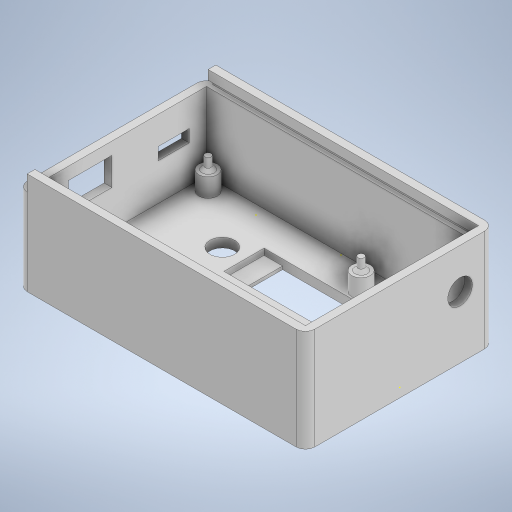
# Autodesk Inventor part: bt-case
Saved by Autodesk Inventor 2024.2 (Build 282272000, 272)
## iProperties
Created: 2025-05-09
Part Number: bt-case
Material: Типовые
Document SubType Name: Modeling
Designer: nikit
Density: 1 g/cm^3
Appearance: По умолчанию
Author: nikit
Autodesk Inventor part; units mm, degrees
ref_plane "YZ Plane" through (0, 0, 0) normal (1, 0, 0) x (0, 1, 0)
ref_plane "XZ Plane" through (0, 0, 0) normal (0, 1, 0) x (-1, 0, 0)
ref_plane "XY Plane" through (0, 0, 0) normal (0, 0, 1) x (1, 0, 0)
sketch "Эскиз1" plane through (0, 0, 0) normal (0, 1, 0) x (-1, 0, 0)
  line L0 (43.5, -27.5) -> (-43.5, -27.5)
  line L1 (-43.5, -27.5) -> (-43.5, 27.5)
  line L2 (-43.5, 27.5) -> (43.5, 27.5)
  line L3 (43.5, 27.5) -> (43.5, -27.5)
  line L4 (43.5, -27.5) -> (-43.5, 27.5) construction
  line L5 (-43.5, -27.5) -> (43.5, 27.5) construction
  arc A0 (46.5, 27.5) -> (43.5, 30.5) centre (43.5, 27.5) ccw
  line L6 (43.5, -30.5) -> (-43.5, -30.5)
  line L7 (-46.5, -27.5) -> (-46.5, 27.5)
  line L8 (-43.5, 30.5) -> (43.5, 30.5)
  line L9 (46.5, 27.5) -> (46.5, -27.5)
  arc A1 (43.5, -30.5) -> (46.5, -27.5) centre (43.5, -27.5) ccw
  arc A2 (-46.5, -27.5) -> (-43.5, -30.5) centre (-43.5, -27.5) ccw
  arc A3 (-43.5, 30.5) -> (-46.5, 27.5) centre (-43.5, 27.5) ccw
  point P0 (0, 0)
  dimension "d0" = 87
  dimension "d1" = 55
  dimension "d4" = 6
  constraints: 20 end point, 8 point on circle, 5 tangent, 4 centre point, 4 coincident, 2 midpoint, 2 parallel, 2 perpendicular, 1 horizontal
  measures "d0" distance of L1.end L2.end
  measures "d1" distance of L0.end L1.end
  measures "d4" diameter of A0
extrude "Выдавливание1" add sketch "Эскиз1" along normal blind 25
sketch "Эскиз2" plane through (0, 0, 0) normal (0, -1, 0) x (1, 0, 0)
  line L0 (43.5, -27.5) -> (43.5, 27.5) projected
  circle A0 centre (43.5, -27.5) radius 3
  line L1 (-43.5, -27.5) -> (43.5, -27.5) projected
  circle A1 centre (-43.5, -27.5) radius 3
  line L2 (43.5, 27.5) -> (-43.5, 27.5) projected
  circle A2 centre (-43.5, 27.5) radius 3
  circle A3 centre (43.5, 27.5) radius 3
  line L3 (-43.5, -30.5) -> (43.5, -30.5)
  line L4 (46.5, 27.5) -> (46.5, -27.5) projected
  line L5 (46.5, -27.5) -> (46.5, 27.5)
  line L6 (-43.5, 30.5) -> (43.5, 30.5) projected
  line L7 (43.5, 30.5) -> (-43.5, 30.5)
  line L8 (-46.5, 27.5) -> (-46.5, -27.5)
  point P0 (0, 0)
  constraints: 8 end point, 5 point on circle, 5 tangent, 4 centre point, 2 collinear, 1 coincident
extrude "Выдавливание2" add sketch "Эскиз2" along normal blind 3
sketch "Эскиз3" plane through (0, 0, 0) normal (0, 1, 0) x (1, 0, 0)
  line L0 (43.5, 27.5) -> (43.5, -27.5) projected
  line L1 (-43.5, 27.5) -> (43.5, 27.5) projected
  line L2 (21.4, 27.5) -> (38.4, 27.5) construction
  circle A0 centre (21.4, 10.5) radius 3.5
  circle A1 centre (21.4, 10.5) radius 4
  point P0 (0, 0)
  dimension "d15" = 8
  constraints: 2 centre point, 2 end point, 1 coincident, 1 horizontal, 1 point on line
  measures "d15" diameter of A1
extrude "Выдавливание3" cut sketch "Эскиз3" against normal blind 86.25 contours A0 | A1
sketch "Эскиз4" plane through (0, 0, 0) normal (0, 1, 0) x (1, 0, 0)
  circle A0 centre (21.4, 10.5) radius 4 projected
  line L0 (21.4, 10.5) -> (14.4, 10.5)
  line L1 (14.4, 10.5) -> (-23.6, 10.5)
  line L2 (14.4, 10.5) -> (8.4, 10.5)
  line L3 (8.4, 10.5) -> (-18.6, 10.5)
  line L4 (8.4, 16.5) -> (-18.6, 16.5)
  line L5 (-18.6, 16.5) -> (-18.6, 4.5)
  line L6 (-18.6, 4.5) -> (8.4, 4.5)
  line L7 (8.4, 4.5) -> (8.4, 16.5)
  line L8 (8.4, 16.5) -> (-18.6, 4.5) construction
  line L9 (-18.6, 16.5) -> (8.4, 4.5) construction
  line L10 (-23.6, 4.5) -> (14.4, 4.5)
  line L11 (14.4, 4.5) -> (14.4, 16.5)
  line L12 (14.4, 16.5) -> (-23.6, 16.5)
  line L13 (-23.6, 16.5) -> (-23.6, 4.5)
  point P0 (0, 0)
  point P1 (-5.1, 10.5)
  dimension "d18" = 7
  dimension "d19" = 38
  dimension "d20" = 6
  dimension "d21" = 27
  dimension "d22" = 12
  constraints: 28 end point, 4 parallel, 3 horizontal, 3 midpoint, 3 point on line, 2 perpendicular
  measures "d18" distance of L0.start L0.end
  measures "d19" distance of L0.end L1.end
  measures "d20" distance of L0.end L2.end
  measures "d21" distance of L2.end L3.end
  measures "d22" distance of L5.end L4.end
extrude "Выдавливание4" cut sketch "Эскиз4" against normal blind 2 contours L11 L10 L7 L1 | L1 L7 L12 L11 | L5 L10 L13 L1 | L1 L13 L12 L5
sketch "Эскиз5" plane through (0, 0, 0) normal (0, 1, 0) x (1, 0, 0)
  line L0 (8.4, 4.5) -> (8.4, 16.5) projected
  line L1 (-23.6, 16.5) -> (-18.6, 16.5) projected
  line L2 (8.4, 4.5) -> (-18.6, 4.5)
  line L3 (-18.6, 4.5) -> (-18.6, 16.5)
  line L4 (-18.6, 16.5) -> (8.4, 16.5)
  line L5 (8.4, 16.5) -> (8.4, 4.5)
  point P0 (0, 0)
  constraints: 8 end point, 2 parallel, 1 horizontal, 1 perpendicular
extrude "Выдавливание5" cut sketch "Эскиз5" against normal blind 3
sketch "Эскиз6" plane through (0, 0, 0) normal (0, 1, 0) x (1, 0, 0)
  point P0 (0, 0)
sketch "Эскиз7" plane through (0, 0, 0) normal (0, 1, 0) x (1, 0, 0)
  line L0 (-43.5, 27.5) -> (43.5, 27.5) projected
  line L1 (43.5, 27.5) -> (39.5, 27.5)
  line L2 (39.5, 27.5) -> (39.5, 24)
  line L3 (39.5, 24) -> (43.5, 24)
  line L4 (43.5, 24) -> (43.5, 27.5)
  circle A0 centre (39.5, 24) radius 3
  line L5 (-43.5, -27.5) -> (-43.5, 27.5) projected
  line L6 (-43.5, -27.5) -> (-39.5, -27.5)
  line L7 (-39.5, -27.5) -> (-39.5, -23)
  line L8 (-39.5, -23) -> (-43.5, -23)
  line L9 (-43.5, -23) -> (-43.5, -27.5)
  circle A1 centre (-39.5, -23) radius 3
  arc A2 (-43.5, 30.5) -> (-46.5, 27.5) centre (-43.5, 27.5) ccw projected
  line L10 (-43.5, 27.5) -> (-13.5, 27.5)
  line L11 (-13.5, 27.5) -> (-13.5, 20.5)
  line L12 (-13.5, 20.5) -> (-43.5, 20.5)
  line L13 (-43.5, 20.5) -> (-43.5, 27.5)
  circle A3 centre (-13.5, 20.5) radius 3
  point P0 (0, 0)
  dimension "d27" = 4
  dimension "d28" = 3.5
  dimension "d29" = 6
  dimension "d30" = 4
  dimension "d31" = 4.5
  dimension "d32" = 6
  dimension "d33" = 30
  dimension "d34" = 7
  dimension "d35" = 6
  constraints: 24 end point, 6 parallel, 3 centre point, 3 coincident, 3 horizontal, 3 perpendicular
  measures "d27" distance of L3.end L2.end
  measures "d28" distance of L2.end L1.end
  measures "d29" diameter of A0
  measures "d30" distance of L8.end L7.end
  measures "d31" distance of L7.end L6.end
  measures "d32" diameter of A1
  measures "d33" distance of L11.end L12.end
  measures "d34" distance of L10.end L11.end
  measures "d35" diameter of A3
extrude "Выдавливание6" add sketch "Эскиз7" along normal blind 6 contours A3 L12 L11 | L11 L12 A3 | A0 L3 L2 | L2 L3 A0 | A1 L7 L8 | L8 L7 A1
sketch "Эскиз8" plane through (39.5, 6, -24) normal (0, 1, 0) x (1, 0, 0)
  circle A0 centre (0, 0) radius 3 projected
  circle A1 centre (0, 0) radius 1
  circle A2 centre (-53, -3.5) radius 3 projected
  circle A3 centre (-53, -3.5) radius 1
  circle A4 centre (-79, -47) radius 3 projected
  circle A5 centre (-79, -47) radius 1
  point P0 (-39.5, -24)
  dimension "d38" = 2
  dimension "d39" = 2
  dimension "d40" = 2
  constraints: 3 centre point, 3 coincident
  measures "d38" diameter of A1
  measures "d39" diameter of A3
  measures "d40" diameter of A5
extrude "Выдавливание7" add sketch "Эскиз8" along normal blind 4 contours A1 | A3 | A5
chamfer "Фаска1" distance 1 angle 45 3 edges at (-40.5, 6, 23) (38.5, 6, -24) (-14.5, 6, -20.5)
sketch "Эскиз9" plane through (-43.5, 25, 27.5) normal (1, 0, 0) x (0, 0, -1)
  point P0 (27.5, -25)
sketch "Эскиз10" plane through (-43.5, 25, 27.5) normal (1, 0, 0) x (0, 0, -1)
  point P0 (27.5, -25)
sketch "Эскиз11" plane through (-43.5, 25, 27.5) normal (1, 0, 0) x (0, 0, -1)
  line L0 (55, 0) -> (55, -28) projected
  line L1 (55, -25) -> (45, -25)
  line L2 (45, -25) -> (45, -15)
  line L3 (45, -15) -> (55, -15)
  line L4 (55, -15) -> (55, -25)
  circle A0 centre (45, -15) radius 6.5
  point P0 (27.5, -25)
  dimension "d54" = 10
  dimension "d55" = 10
  dimension "d56" = 13
  constraints: 8 end point, 2 parallel, 1 centre point, 1 coincident, 1 horizontal, 1 perpendicular, 1 point on line
  measures "d54" distance of L2.end L3.end
  measures "d55" distance of L1.end L2.end
  measures "d56" diameter of A0
extrude "Выдавливание8" cut sketch "Эскиз11" against normal blind 5.75 contours A0 L2 L3 | L3 L2 A0
sketch "Эскиз12" plane through (46.5, 25, 27.5) normal (1, 0, 0) x (0, 0, -1)
  line L0 (-3, -28) -> (0, -28) projected
  line L1 (0, -28) -> (0, -25)
  line L2 (0, -28) -> (0, 0) projected
  line L3 (0, -25) -> (0, -17)
  line L4 (6.5, -19) -> (2.5, -19) projected
  line L5 (14.25, -17) -> (14.25, -20.5)
  line L6 (5, -20.5) -> (23.5, -20.5)
  line L7 (23.5, -20.5) -> (23.5, -17)
  line L8 (5, -17) -> (5, -20.5)
  line L9 (5, -20.5) -> (23.5, -17) construction
  line L10 (23.5, -20.5) -> (5, -17) construction
  line L11 (5, -17) -> (23.5, -17)
  point P0 (27.5, -25)
  point P1 (14.25, -18.75)
  dimension "d72" = 3.5
  dimension "d73" = 18.5
  constraints: 18 end point, 3 midpoint, 2 horizontal, 2 point on line, 1 parallel, 1 perpendicular, 1 vertical
  measures "d72" distance of L5.start L5.end
  measures "d73" distance of L6.start L6.end
extrude "Выдавливание9" cut sketch "Эскиз12" against normal blind 4.25
sketch "Эскиз13" plane through (0, 25, 0) normal (0, 1, 0) x (1, 0, 0)
  point P0 (0, 0)
sketch "Эскиз14" plane through (0, 25, 0) normal (0, 1, 0) x (1, 0, 0)
  line L0 (-43.5, 27.5) -> (43.5, 27.5) projected
  line L1 (43.5, 27.5) -> (-43.5, 27.5)
  line L2 (-43.5, 27.5) -> (-43.5, -27.5)
  line L3 (-43.5, -27.5) -> (43.5, -27.5)
  arc A0 (46.5, 27.5) -> (43.5, 30.5) centre (43.5, 27.5) ccw projected
  line L4 (43.5, 27.5) -> (43.5, 30.5)
  line L5 (43.5, 30.5) -> (-43.5, 30.5)
  arc A1 (-46.5, -27.5) -> (-43.5, -30.5) centre (-43.5, -27.5) ccw projected
  line L6 (-43.5, -30.5) -> (43.5, -30.5)
  line L7 (43.5, -30.5) -> (43.5, -27.5)
  arc A2 (-46.5, -27.5) -> (-43.5, -30.5) centre (-43.5, -27.5) ccw
  arc A3 (-43.5, 30.5) -> (-46.5, 27.5) centre (-43.5, 27.5) ccw projected
  arc A4 (-43.5, 30.5) -> (-46.5, 27.5) centre (-43.5, 27.5) ccw
  line L8 (-46.5, 27.5) -> (-46.5, -27.5)
  point P0 (0, 0)
  constraints: 16 end point, 5 point on circle, 5 tangent, 4 perpendicular, 2 centre point, 2 vertical, 1 collinear, 1 horizontal
extrude "Выдавливание10" add sketch "Эскиз14" along normal blind 5
sketch "Эскиз15" plane through (43.5, 25, 30.5) normal (1, 0, 0) x (0, 0, -1)
  line L0 (3, 0) -> (3, 5) projected
  line L1 (3, 0) -> (1, 0)
  line L2 (1, 0) -> (1, 2)
  line L3 (1, 2) -> (3, 2)
  line L4 (3, 2) -> (3, 0)
  line L5 (61, 0) -> (58, 0) projected
  line L6 (58, 0) -> (60, 0)
  line L7 (60, 0) -> (60, 2)
  line L8 (60, 2) -> (58, 2)
  line L9 (58, 2) -> (58, 0)
  point P0 (30.5, -25)
  point P1 (3, 2)
  dimension "d78" = 2
  dimension "d79" = 2
  dimension "d80" = 2
  dimension "d81" = 2
  constraints: 16 end point, 4 parallel, 2 horizontal, 2 perpendicular
  measures "d78" distance of L2.end L3.end
  measures "d79" distance of L1.end L2.end
  measures "d80" distance of L8.end L7.end
  measures "d81" distance of L7.end L6.end
extrude "Выдавливание11" cut sketch "Эскиз15" against normal blind 87
mirror "Зеркальное отражение1" about plane through (0, 0, 0) normal (1, 0, 0) remove original yes
sketch "Эскиз16" plane through (-43.5, 0, -27.5) normal (0, 1, 0) x (1, 0, 0)
  line L0 (29.1, -11) -> (29.1, -23) projected
  line L1 (29.1, -11) -> (29.1, -10.5)
  line L2 (62.1, -23) -> (67.1, -23) projected
  line L3 (67.1, -23) -> (67.1, -23.5)
  line L4 (29.1, -10.5) -> (67.1, -10.5)
  line L5 (67.1, -10.5) -> (67.1, -23.5)
  line L6 (67.1, -23.5) -> (29.1, -23.5)
  line L7 (29.1, -23.5) -> (29.1, -10.5)
  point P0 (43.5, -27.5)
  dimension "d84" = 0.5
  dimension "d85" = 0.5
  constraints: 12 end point, 2 parallel, 2 vertical, 1 horizontal, 1 perpendicular
  measures "d84" distance of L0.start L1.end
  measures "d85" distance of L2.end L3.end
extrude "Выдавливание12" cut sketch "Эскиз16" against normal blind 2
sketch "Эскиз17" plane through (-14.4, -2, -17) normal (0, 1, 0) x (1, 0, 0)
  line L0 (6, -0.5) -> (33, -0.5) projected
  line L1 (6, -0.5) -> (6, 0)
  line L2 (0, 0) -> (38, 0) projected
  line L3 (33, -0.5) -> (33, -12.5) projected
  line L4 (33, -12.5) -> (33, -13)
  line L5 (38, -13) -> (0, -13) projected
  line L6 (6, 0) -> (33, 0)
  line L7 (33, 0) -> (33, -13)
  line L8 (33, -13) -> (6, -13)
  line L9 (6, -13) -> (6, 0)
  point P0 (14.4, -17)
  constraints: 12 end point, 2 parallel, 2 point on line, 2 vertical, 1 horizontal, 1 perpendicular
extrude "Выдавливание13" cut sketch "Эскиз17" against normal blind 2
sketch "Эскиз18" plane through (46.5, -3, 27.5) normal (1, 0, 0) x (0, 0, -1)
  circle A0 centre (45, 13) radius 6.5 projected
  circle A1 centre (45, 13) radius 6.5
  point P0 (27.5, 3)
  constraints: 1 centre point, 1 coincident
extrude "Выдавливание14" add sketch "Эскиз18" against normal blind 3
sketch "Эскиз19" plane through (46.5, -3, 27.5) normal (1, 0, 0) x (0, 0, -1)
  point P0 (27.5, 3)
sketch "Эскиз20" plane through (46.5, -3, 27.5) normal (1, 0, 0) x (0, 0, -1)
  line L0 (55, 0) -> (0, 0) projected
  line L1 (47, 0) -> (47, 20)
  line L2 (47, 0) -> (67, 0) construction
  circle A0 centre (47, 20) radius 4
  line L3 (55, 33) -> (55, 0) projected
  point P0 (27.5, 3)
  dimension "d92" = 20
  dimension "d93" = 90
  dimension "d94" = 8
  dimension "d95" = 8
  constraints: 4 end point, 2 perpendicular, 1 centre point, 1 coincident, 1 horizontal, 1 point on line
  measures "d92" distance of L1.start L1.end
  measures "d93" angle of L2 L1
  measures "d94" diameter of A0
  measures "d95" distance from line of L3 A0.centre
extrude "Выдавливание15" cut sketch "Эскиз20" against normal blind 23.75
sketch "Эскиз21" plane through (-46.5, -3, -27.5) normal (-1, 0, 0) x (0, 0, 1)
  line L0 (50, 11) -> (31.5, 11) projected
  line L1 (50, 7.5) -> (31.5, 7.5) projected
  line L2 (31.5, 11) -> (50, 11)
  line L3 (50, 11) -> (50, 7.5)
  line L4 (50, 7.5) -> (31.5, 7.5)
  line L5 (31.5, 7.5) -> (31.5, 11)
  point P0 (27.5, 3)
  constraints: 8 end point, 2 parallel, 1 horizontal, 1 perpendicular
extrude "Выдавливание16" add sketch "Эскиз21" against normal blind 3
sketch "Эскиз22" plane through (-46.5, -3, -27.5) normal (-1, 0, 0) x (0, 0, 1)
  line L0 (0, 0) -> (55, 0) projected
  line L1 (5.1274, 0) -> (5.1274, 15)
  line L2 (5.1274, 0) -> (20.1274, 0) construction
  line L3 (5.1274, 15) -> (5.1274, 19)
  line L4 (5.1274, 19) -> (15.1274, 19)
  line L5 (15.1274, 19) -> (15.1274, 15)
  line L6 (15.1274, 15) -> (5.1274, 15)
  line L7 (5.1274, 15) -> (5.1274, 19)
  line L8 (15.1274, 15) -> (30.1274, 15)
  line L9 (15.1274, 15) -> (30.1274, 15) construction
  line L10 (30.1274, 15) -> (44.1274, 15)
  line L11 (44.1274, 15) -> (44.1274, 24)
  line L12 (44.1274, 24) -> (30.1274, 24)
  line L13 (30.1274, 24) -> (30.1274, 15)
  point P0 (27.5, 3)
  point P1 (5.1274, 15)
  dimension "d100" = 15
  dimension "d101" = 90
  dimension "d102" = 4
  dimension "d103" = 10
  dimension "d104" = 4
  dimension "d105" = 15
  dimension "d107" = 14
  dimension "d108" = 9
  constraints: 26 end point, 5 horizontal, 4 parallel, 3 perpendicular, 2 equal length, 1 point on line, 1 vertical
  measures "d100" distance of L1.start L1.end
  measures "d101" angle of L2 L1
  measures "d102" distance of L1.end L3.end
  measures "d103" distance of L5.end L6.end
  measures "d104" distance of L4.end L5.end
  measures "d105" distance of L5.end L8.end
  measures "d107" distance of L12.end L11.end
  measures "d108" distance of L11.end L10.end
extrude "Выдавливание17" cut sketch "Эскиз22" against normal blind 3
sketch "Эскиз23" plane through (-43.5, 0, -27.5) normal (0, 0, 1) x (1, 0, 0)
  point P0 (43.5, 0)
sketch "Эскиз24" plane through (-43.5, 0, -27.5) normal (0, 0, 1) x (1, 0, 0)
  line L0 (0, 0) -> (0, 25) projected
  line L1 (87, 30) -> (0, 30) projected
  line L2 (0, 0) -> (87, 0)
  line L3 (87, 0) -> (87, 30)
  line L4 (87, 30) -> (0, 30)
  line L5 (0, 30) -> (0, 0)
  point P0 (43.5, 0)
  constraints: 8 end point, 2 parallel, 1 horizontal, 1 perpendicular
extrude "Выдавливание18" cut sketch "Эскиз24" against normal blind 0.5
sketch "Эскиз25" plane through (43.5, 0, 27.5) normal (0, 0, -1) x (-1, 0, 0)
  line L0 (87, 0) -> (0, 0) projected
  line L1 (0, 0) -> (87, 0)
  line L2 (87, 0) -> (87, 30)
  line L3 (87, 30) -> (0, 30)
  line L4 (0, 30) -> (0, 0)
  point P0 (43.5, 0)
  constraints: 8 end point, 2 parallel, 1 horizontal, 1 perpendicular
extrude "Выдавливание19" cut sketch "Эскиз25" against normal blind 0.5
sketch "Эскиз26" plane through (43.5, 25, -29.5) normal (-1, 0, 0) x (0, 0, 1)
  line L0 (1.5, 0) -> (1.5, -25) projected
  line L1 (1.5, 5) -> (57.5, 5) projected
  line L2 (1.5, -25) -> (57.5, -25)
  line L3 (57.5, -25) -> (57.5, 5)
  line L4 (57.5, 5) -> (1.5, 5)
  line L5 (1.5, 5) -> (1.5, -25)
  point P0 (29.5, -25)
  constraints: 8 end point, 2 parallel, 1 horizontal, 1 perpendicular
extrude "Выдавливание20" cut sketch "Эскиз26" against normal blind 0.5
sketch "Эскиз27" plane through (-43.5, 0, -28) normal (1, 0, 0) x (0, 0, -1)
  line L0 (-56, 25) -> (-56, 0) projected
  line L1 (0, 0) -> (0, 25) projected
  line L2 (-56, 0) -> (0, 0)
  line L3 (0, 0) -> (0, 25)
  line L4 (0, 25) -> (-56, 25)
  line L5 (-56, 25) -> (-56, 0)
  point P0 (-28, 0)
  constraints: 8 end point, 2 parallel, 1 horizontal, 1 perpendicular
extrude "Выдавливание21" cut sketch "Эскиз27" against normal blind 0.5
